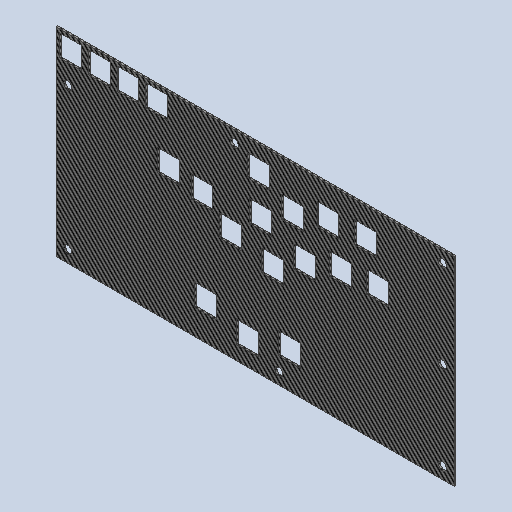
# Autodesk Inventor part: Positioning_Plate
Saved by Autodesk Inventor 2024 (Build 280153000, 153)
## iProperties
Created: 2023-09-20
Part Number: Positioning_Plate
Material: 常规
Document SubType Name: Modeling
Designer: nicx5
Density: 1 g/cm^3
Appearance: 碳纤维
Author: nicx5
Autodesk Inventor part; units mm, degrees
ref_plane "YZ Plane" through (0, 0, 0) normal (1, 0, 0) x (0, 1, 0)
ref_plane "XZ Plane" through (0, 0, 0) normal (0, 1, 0) x (-1, 0, 0)
ref_plane "XY Plane" through (0, 0, 0) normal (0, 0, 1) x (1, 0, 0)
derived "Frame.ipt"
sketch "定位板草图" plane through (0, 0, -7) normal (0, 0, 1) x (1, 0, 0)
  line L0 (128, -53) -> (128, 75)
  line L1 (128, 75) -> (-128, 75)
  line L2 (-128, 75) -> (-128, -53)
  line L3 (-128, -53) -> (128, -53)
  line L4 (-55.7514, 33.4183) -> (-34.0856, 29.598)
  line L5 (-34.0856, 29.598) -> (-16.0643, 16.9793)
  line L6 (2.0127, 59.4994) -> (3.7009, 34.6338)
  line L7 (3.7009, 34.6338) -> (24.0951, 47.2859)
  line L8 (24.0951, 47.2859) -> (46.9166, 54.7144)
  line L9 (46.9166, 54.7144) -> (70.8507, 56.4914)
  line L10 (54.6939, 31.0574) -> (78.628, 32.8344)
  line L11 (31.8725, 23.629) -> (54.6939, 31.0574)
  line L12 (11.4783, 10.9768) -> (31.8725, 23.629)
  line L13 (-5.0643, -36.9094) -> (21.9949, -29.7121)
  line L14 (-32.1234, -29.7121) -> (-5.0643, -36.9094)
  line L15 (-62.7764, 40.4433) -> (-48.7264, 40.4433)
  line L16 (-48.7264, 40.4433) -> (-48.7264, 26.3933)
  line L17 (-48.7264, 26.3933) -> (-62.7764, 26.3933)
  line L18 (-62.7764, 26.3933) -> (-62.7764, 40.4433)
  line L19 (-62.7764, 40.4433) -> (-48.7264, 26.3933)
  line L20 (-48.7264, 40.4433) -> (-62.7764, 26.3933)
  line L21 (-41.1106, 36.623) -> (-27.0606, 36.623)
  line L22 (-27.0606, 36.623) -> (-27.0606, 22.573)
  line L23 (-27.0606, 22.573) -> (-41.1106, 22.573)
  line L24 (-41.1106, 22.573) -> (-41.1106, 36.623)
  line L25 (-41.1106, 36.623) -> (-27.0606, 22.573)
  line L26 (-27.0606, 36.623) -> (-41.1106, 22.573)
  line L27 (-23.0893, 24.0043) -> (-9.0393, 24.0043)
  line L28 (-9.0393, 24.0043) -> (-9.0393, 9.9543)
  line L29 (-9.0393, 9.9543) -> (-23.0893, 9.9543)
  line L30 (-23.0893, 9.9543) -> (-23.0893, 24.0043)
  line L31 (-23.0893, 24.0043) -> (-9.0393, 9.9543)
  line L32 (-9.0393, 24.0043) -> (-23.0893, 9.9543)
  line L33 (-39.1484, -22.6871) -> (-25.0984, -22.6871)
  line L34 (-25.0984, -22.6871) -> (-25.0984, -36.7371)
  line L35 (-25.0984, -36.7371) -> (-39.1484, -36.7371)
  line L36 (-39.1484, -36.7371) -> (-39.1484, -22.6871)
  line L37 (-39.1484, -22.6871) -> (-25.0984, -36.7371)
  line L38 (-25.0984, -22.6871) -> (-39.1484, -36.7371)
  line L39 (-12.0893, -29.8844) -> (1.9607, -29.8844)
  line L40 (1.9607, -29.8844) -> (1.9607, -43.9344)
  line L41 (1.9607, -43.9344) -> (-12.0893, -43.9344)
  line L42 (-12.0893, -43.9344) -> (-12.0893, -29.8844)
  line L43 (-12.0893, -29.8844) -> (1.9607, -43.9344)
  line L44 (1.9607, -29.8844) -> (-12.0893, -43.9344)
  line L45 (14.9699, -22.6871) -> (29.0199, -22.6871)
  line L46 (29.0199, -22.6871) -> (29.0199, -36.7371)
  line L47 (29.0199, -36.7371) -> (14.9699, -36.7371)
  line L48 (14.9699, -36.7371) -> (14.9699, -22.6871)
  line L49 (14.9699, -22.6871) -> (29.0199, -36.7371)
  line L50 (29.0199, -22.6871) -> (14.9699, -36.7371)
  line L51 (4.4533, 18.0018) -> (18.5033, 18.0018)
  line L52 (18.5033, 18.0018) -> (18.5033, 3.9518)
  line L53 (18.5033, 3.9518) -> (4.4533, 3.9518)
  line L54 (4.4533, 3.9518) -> (4.4533, 18.0018)
  line L55 (4.4533, 18.0018) -> (18.5033, 3.9518)
  line L56 (18.5033, 18.0018) -> (4.4533, 3.9518)
  line L57 (24.8475, 30.654) -> (38.8975, 30.654)
  line L58 (38.8975, 30.654) -> (38.8975, 16.604)
  line L59 (38.8975, 16.604) -> (24.8475, 16.604)
  line L60 (24.8475, 16.604) -> (24.8475, 30.654)
  line L61 (24.8475, 30.654) -> (38.8975, 16.604)
  line L62 (38.8975, 30.654) -> (24.8475, 16.604)
  line L63 (47.6689, 38.0824) -> (61.7189, 38.0824)
  line L64 (61.7189, 38.0824) -> (61.7189, 24.0324)
  line L65 (61.7189, 24.0324) -> (47.6689, 24.0324)
  line L66 (47.6689, 24.0324) -> (47.6689, 38.0824)
  line L67 (47.6689, 38.0824) -> (61.7189, 24.0324)
  line L68 (61.7189, 38.0824) -> (47.6689, 24.0324)
  line L69 (71.603, 39.8594) -> (85.653, 39.8594)
  line L70 (85.653, 39.8594) -> (85.653, 25.8094)
  line L71 (85.653, 25.8094) -> (71.603, 25.8094)
  line L72 (71.603, 25.8094) -> (71.603, 39.8594)
  line L73 (71.603, 39.8594) -> (85.653, 25.8094)
  line L74 (85.653, 39.8594) -> (71.603, 25.8094)
  line L75 (-3.3241, 41.6588) -> (10.7259, 41.6588)
  line L76 (10.7259, 41.6588) -> (10.7259, 27.6088)
  line L77 (10.7259, 27.6088) -> (-3.3241, 27.6088)
  line L78 (-3.3241, 27.6088) -> (-3.3241, 41.6588)
  line L79 (-3.3241, 41.6588) -> (10.7259, 27.6088)
  line L80 (10.7259, 41.6588) -> (-3.3241, 27.6088)
  line L81 (17.0701, 54.3109) -> (31.1201, 54.3109)
  line L82 (31.1201, 54.3109) -> (31.1201, 40.2609)
  line L83 (31.1201, 40.2609) -> (17.0701, 40.2609)
  line L84 (17.0701, 40.2609) -> (17.0701, 54.3109)
  line L85 (17.0701, 54.3109) -> (31.1201, 40.2609)
  line L86 (31.1201, 54.3109) -> (17.0701, 40.2609)
  line L87 (39.8916, 61.7394) -> (53.9416, 61.7394)
  line L88 (53.9416, 61.7394) -> (53.9416, 47.6894)
  line L89 (53.9416, 47.6894) -> (39.8916, 47.6894)
  line L90 (39.8916, 47.6894) -> (39.8916, 61.7394)
  line L91 (39.8916, 61.7394) -> (53.9416, 47.6894)
  line L92 (53.9416, 61.7394) -> (39.8916, 47.6894)
  line L93 (63.8257, 63.5164) -> (77.8757, 63.5164)
  line L94 (77.8757, 63.5164) -> (77.8757, 49.4664)
  line L95 (77.8757, 49.4664) -> (63.8257, 49.4664)
  line L96 (63.8257, 49.4664) -> (63.8257, 63.5164)
  line L97 (63.8257, 63.5164) -> (77.8757, 49.4664)
  line L98 (77.8757, 63.5164) -> (63.8257, 49.4664)
  line L99 (-5.0123, 66.5244) -> (9.0377, 66.5244)
  line L100 (9.0377, 66.5244) -> (9.0377, 52.4744)
  line L101 (9.0377, 52.4744) -> (-5.0123, 52.4744)
  line L102 (-5.0123, 52.4744) -> (-5.0123, 66.5244)
  line L103 (-5.0123, 66.5244) -> (9.0377, 52.4744)
  line L104 (9.0377, 66.5244) -> (-5.0123, 52.4744)
  line L105 (-127.5039, 40.0108) -> (-74.5039, 40.0108)
  line L106 (-74.5039, 40.0108) -> (-74.5039, 17.0108)
  line L107 (-74.5039, 17.0108) -> (-127.5039, 17.0108)
  line L108 (-127.5039, 17.0108) -> (-127.5039, 40.0108)
  line L109 (-128, 75) -> (-109.5, 56.5)
  line L110 (-109.5, 75) -> (-91, 56.5)
  line L111 (-91, 75) -> (-72.5, 56.5)
  line L112 (-72.5, 75) -> (-54, 56.5)
  line L113 (-125.775, 72.775) -> (-111.725, 72.775)
  line L114 (-111.725, 72.775) -> (-111.725, 58.725)
  line L115 (-111.725, 58.725) -> (-125.775, 58.725)
  line L116 (-125.775, 58.725) -> (-125.775, 72.775)
  line L117 (-125.775, 72.775) -> (-111.725, 58.725)
  line L118 (-111.725, 72.775) -> (-125.775, 58.725)
  line L119 (-107.275, 72.775) -> (-93.225, 72.775)
  line L120 (-93.225, 72.775) -> (-93.225, 58.725)
  line L121 (-93.225, 58.725) -> (-107.275, 58.725)
  line L122 (-107.275, 58.725) -> (-107.275, 72.775)
  line L123 (-107.275, 72.775) -> (-93.225, 58.725)
  line L124 (-93.225, 72.775) -> (-107.275, 58.725)
  line L125 (-88.775, 72.775) -> (-74.725, 72.775)
  line L126 (-74.725, 72.775) -> (-74.725, 58.725)
  line L127 (-74.725, 58.725) -> (-88.775, 58.725)
  line L128 (-88.775, 58.725) -> (-88.775, 72.775)
  line L129 (-88.775, 72.775) -> (-74.725, 58.725)
  line L130 (-74.725, 72.775) -> (-88.775, 58.725)
  line L131 (-70.275, 72.775) -> (-56.225, 72.775)
  line L132 (-56.225, 72.775) -> (-56.225, 58.725)
  line L133 (-56.225, 58.725) -> (-70.275, 58.725)
  line L134 (-70.275, 58.725) -> (-70.275, 72.775)
  line L135 (-70.275, 72.775) -> (-56.225, 58.725)
  line L136 (-56.225, 72.775) -> (-70.275, 58.725)
  circle A0 centre (-120.5, 46) radius 1.275
  circle A1 centre (-120.5, -45.5) radius 1.275
  circle A2 centre (15.3724, -45.5) radius 1.275
  circle A3 centre (120.5, -45.5) radius 1.275
  circle A4 centre (120.5, 11) radius 1.275
  circle A5 centre (120.5, 67.5) radius 1.275
  circle A6 centre (-13.3354, 67.5) radius 1.275
  circle A7 centre (120.5, 67.5) radius 4
  circle A8 centre (-13.3354, 67.5) radius 4
  circle A9 centre (120.5, 11) radius 4
  circle A10 centre (120.5, -45.5) radius 4
  circle A11 centre (15.3724, -45.5) radius 4
  circle A12 centre (-120.5, -45.5) radius 4
  circle A13 centre (-120.5, 46) radius 4
  point P0 (-118.75, 65.75)
  point P1 (-100.25, 65.75)
  point P2 (-81.75, 65.75)
  point P3 (-63.25, 65.75)
extrude "拉伸1" add sketch "定位板草图" along normal blind 1.2 contours L3 L2 L1 L0 | L105 L106 L107 L108 | A0 | A1 | A2 | A3 | A4 | A5 | A6 | A7 | A8 | A9 | A10 | A11 | A12 | A13
hole "孔1" at (120.5, 67.5, -7) at (120.5, 11, -7) at (120.5, -45.5, -7) at (15.3724, -45.5, -7) at (-13.3354, 67.5, -7) at (-120.5, 46, -7) at (-120.5, -45.5, -7) direction (0, 0, 1) diameter 5.2 end through all
